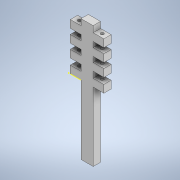
# Autodesk Inventor part: Center
Saved by Autodesk Inventor 2020 (Build 240168000, 168)
## iProperties
Created: 2020-03-31
Part Number: Center
Material: Generic
Document SubType Name: Modeling
Designer: Sverrir
Density: 1 g/cm^3
Appearance: Default
Author: Sverrir
Autodesk Inventor part; units mm, degrees
ref_plane "YZ Plane" through (0, 0, 0) normal (1, 0, 0) x (0, 1, 0)
ref_plane "XZ Plane" through (0, 0, 0) normal (0, 1, 0) x (-1, 0, 0)
ref_plane "Work Plane1" through (40, -59.8973, -11.9951) normal (0, 0, -1) x (0, 1, 0)
sketch "Sketch1" plane through (0, 0, 0) normal (0, 0, 1) x (1, 0, 0)
  line L0 (2.5, -40.193) -> (20, -40.193) projected
  line L1 (20, -31.5948) -> (20, -40.193) projected
  line L2 (20, -31.5948) -> (2.5, -31.5948) projected
  line L3 (2.5, -31.5948) -> (2.5, -19.0948) projected
  line L4 (2.5, -19.0948) -> (20, -19.0948) projected
  line L5 (20, -10.4966) -> (20, -19.0948) projected
  line L6 (20, -10.4966) -> (2.5, -10.4966) projected
  line L7 (2.5, -10.4966) -> (2.5, 2.0034) projected
  line L8 (2.5, 2.0034) -> (20, 2.0034) projected
  line L9 (20, 12.0034) -> (20, 2.0034) projected
  line L10 (-7.708, 12.0034) -> (20, 12.0034) projected
  line L11 (-7.708, -62.693) -> (-7.708, 12.0034) projected
  line L12 (-7.708, -62.693) -> (20, -62.693) projected
  line L13 (20, -52.693) -> (20, -62.693) projected
  line L14 (20, -52.693) -> (2.5, -52.693) projected
  line L15 (2.5, -52.693) -> (2.5, -40.193) projected
  line L16 (57.5, -10.4966) -> (40, -10.4966) projected
  line L17 (40, -19.0948) -> (40, -10.4966) projected
  line L18 (40, -19.0948) -> (57.5, -19.0948) projected
  line L19 (57.5, -19.0948) -> (57.5, -31.5948) projected
  line L20 (57.5, -31.5948) -> (40, -31.5948) projected
  line L21 (40, -40.193) -> (40, -31.5948) projected
  line L22 (40, -40.193) -> (57.5, -40.193) projected
  line L23 (57.5, -40.193) -> (57.5, -52.693) projected
  line L24 (57.5, -52.693) -> (40, -52.693) projected
  line L25 (40, -62.693) -> (40, -52.693) projected
  line L26 (67.708, -62.693) -> (40, -62.693) projected
  line L27 (67.708, 12.0034) -> (67.708, -62.693) projected
  line L28 (67.708, 12.0034) -> (40, 12.0034) projected
  line L29 (40, 2.0034) -> (40, 12.0034) projected
  line L30 (40, 2.0034) -> (57.5, 2.0034) projected
  line L31 (57.5, 2.0034) -> (57.5, -10.4966) projected
  line L32 (20, 12.0034) -> (40, 12.0034)
  line L33 (40, -187.9966) -> (20, -187.9966)
  line L34 (57.5, -62.693) -> (57.5, -75.193)
  line L35 (57.5, -75.193) -> (40, -75.193)
  line L36 (40, -75.193) -> (40, -187.9966)
  line L37 (2.5, -62.693) -> (2.5, -75.193)
  line L38 (2.5, -75.193) -> (20, -75.193)
  line L39 (20, -75.193) -> (20, -187.9966)
  point P0 (0, 0)
  dimension "d0" = 200
  dimension "d1" = 17.5
  dimension "d2" = 17.5
  dimension "d3" = 12.5
  constraints: 16 end point, 3 perpendicular, 3 point on line, 2 horizontal, 2 vertical, 1 collinear, 1 parallel
  measures "d0" distance between parallel lines of L33 L32
  measures "d1" distance between parallel lines of L25 L34
  measures "d2" distance between parallel lines of L13 L37
  measures "d3" distance between parallel lines of L12 L38
extrude "Extrusion1" add sketch "Sketch1" against normal up to surface (11.9951 mm away) contours L0 L1 L2 L3 L4 L5 L6 L7 L8 L9 L32 L29 L30 L31 L16 L17 L18 L19 L20 L21 L22 L23 L24 L25 L26 L34 L35 L36 L33 L39 L38 L37 L12 L13 L14 L15
sketch "Sketch2" plane through (2.5, -75.193, 0) normal (0, -1, 0) x (1, 0, 0)
  line L0 (0, -11.9951) -> (17.5, -11.9951) projected
  line L1 (17.5, 0) -> (17.5, -11.9951) projected
  line L2 (0, 0) -> (17.5, 0) projected
  line L3 (0, 0) -> (0, -11.9951) projected
  line L4 (0, 0) -> (17.5, 0) projected
  line L5 (17.5, 0) -> (17.5, -11.9951) projected
  line L6 (0, 0) -> (17.5, -11.9951)
  circle A0 centre (10, -6.6174) radius 3.3205
  point P0 (-2.5, 0)
  constraints: 2 end point, 1 centre point
sketch "Sketch3" plane through (2.5, 2.0034, 0) normal (0, 1, 0) x (1, 0, 0)
  circle A0 centre (8.75, 5.9976) radius 2.5 projected
  circle A1 centre (8.75, 5.9976) radius 2.5 projected
  line L0 (0, 0) -> (17.5, 0) projected
  line L1 (17.5, 0) -> (17.5, 11.9951) construction
  line L2 (0, 0) -> (17.5, 11.9951) construction
  line L3 (17.5, 11.9951) -> (0, 11.9951) construction
  line L4 (0, 11.9951) -> (17.5, 0) construction
  line L5 (37.5, 0) -> (37.5, 11.9951) construction
  line L6 (37.5, 11.9951) -> (55, 11.9951) construction
  line L7 (37.5, 0) -> (55, 11.9951) construction
  line L8 (55, 11.9951) -> (37.5, 11.9951) construction
  line L9 (37.5, 11.9951) -> (55, 0) construction
  circle A2 centre (46.25, 5.9976) radius 2.5
  point P0 (-2.5, 0)
  dimension "d7" = 5
  constraints: 12 end point, 1 centre point, 1 collinear, 1 midpoint, 1 perpendicular
  measures "d7" diameter of A2
extrude "Extrusion2" cut sketch "Sketch3" against normal blind 86.2
body "Solid1"
